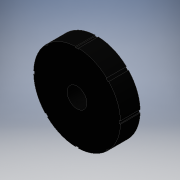
# Autodesk Inventor part: ET2
Saved by Autodesk Inventor 2016 (Build 200138000, 138)
## iProperties
Created: 2016-03-19
Part Number: ET2
Material: Genérico
Document SubType Name: Modeling
Designer: Usuario1
Density: 1 g/cm^3
Appearance: Valor por defecto
Author: Usuario1
Autodesk Inventor part; units mm, degrees
ref_plane "YZ Plane" through (0, 0, 0) normal (1, 0, 0) x (0, 1, 0)
ref_plane "XZ Plane" through (0, 0, 0) normal (0, 1, 0) x (-1, 0, 0)
ref_plane "XY Plane" through (0, 0, 0) normal (0, 0, 1) x (1, 0, 0)
sketch "Boceto1" plane through (0, 0, 0) normal (0, 1, 0) x (-1, 0, 0)
  circle A0 centre (0, 0) radius 0.2442
  circle A1 centre (0, 0) radius 0.28
  line L0 (-0.03, -0.8791) -> (-0.03, -0.8595)
  line L1 (-0.03, -0.8595) -> (0.03, -0.8595)
  line L2 (0.03, -0.8595) -> (0.03, -0.8791)
  line L3 (-0.6428, -0.6004) -> (-0.629, -0.5865)
  line L4 (-0.629, -0.5865) -> (-0.5865, -0.629)
  line L5 (-0.5865, -0.629) -> (-0.6004, -0.6428)
  line L6 (-0.8791, -0.03) -> (-0.8595, -0.03)
  line L7 (-0.8595, -0.03) -> (-0.8595, 0.03)
  line L8 (-0.8595, 0.03) -> (-0.8791, 0.03)
  arc A2 (-0.8791, -0.03) -> (-0.6428, -0.6004) centre (0, 0) ccw
  arc A3 (-0.6004, -0.6428) -> (-0.03, -0.8791) centre (0, 0) ccw
  line L9 (0.03, -0.8791) -> (0.03, -0.8595)
  line L10 (0.03, -0.8595) -> (-0.03, -0.8595)
  line L11 (-0.03, -0.8595) -> (-0.03, -0.8791)
  line L12 (0.6428, -0.6004) -> (0.629, -0.5865)
  line L13 (0.629, -0.5865) -> (0.5865, -0.629)
  line L14 (0.5865, -0.629) -> (0.6004, -0.6428)
  line L15 (0.8791, -0.03) -> (0.8595, -0.03)
  line L16 (0.8595, -0.03) -> (0.8595, 0.03)
  line L17 (0.8595, 0.03) -> (0.8791, 0.03)
  arc A4 (0.6428, -0.6004) -> (0.8791, -0.03) centre (0, 0) ccw
  arc A5 (0.03, -0.8791) -> (0.6004, -0.6428) centre (0, 0) ccw
  line L18 (-0.03, 0.8791) -> (-0.03, 0.8595)
  line L19 (-0.03, 0.8595) -> (0.03, 0.8595)
  line L20 (0.03, 0.8595) -> (0.03, 0.8791)
  line L21 (-0.6428, 0.6004) -> (-0.629, 0.5865)
  line L22 (-0.629, 0.5865) -> (-0.5865, 0.629)
  line L23 (-0.5865, 0.629) -> (-0.6004, 0.6428)
  line L24 (-0.8791, 0.03) -> (-0.8595, 0.03)
  line L25 (-0.8595, 0.03) -> (-0.8595, -0.03)
  line L26 (-0.8595, -0.03) -> (-0.8791, -0.03)
  arc A6 (-0.6428, 0.6004) -> (-0.8791, 0.03) centre (0, 0) ccw
  arc A7 (-0.03, 0.8791) -> (-0.6004, 0.6428) centre (0, 0) ccw
  line L27 (0.03, 0.8791) -> (0.03, 0.8595)
  line L28 (0.03, 0.8595) -> (-0.03, 0.8595)
  line L29 (-0.03, 0.8595) -> (-0.03, 0.8791)
  line L30 (0.6428, 0.6004) -> (0.629, 0.5865)
  line L31 (0.629, 0.5865) -> (0.5865, 0.629)
  line L32 (0.5865, 0.629) -> (0.6004, 0.6428)
  line L33 (0.8791, 0.03) -> (0.8595, 0.03)
  line L34 (0.8595, 0.03) -> (0.8595, -0.03)
  line L35 (0.8595, -0.03) -> (0.8791, -0.03)
  arc A8 (0.8791, 0.03) -> (0.6428, 0.6004) centre (0, 0) ccw
  arc A9 (0.6004, 0.6428) -> (0.03, 0.8791) centre (0, 0) ccw
  circle A10 centre (0, 0) radius 0.2
  point P0 (0, 0)
  constraints: 72 end point, 16 point on circle, 11 centre point
extrude "Extrusión1" add sketch "Boceto1" along normal blind 0.4 contours A0 | A1 | A3 L5 L4 L3 A2 L6 L7 L8 A6 L21 L22 L23 A7 L18 L19 L20 A9 L32 L31 L30 A8 L17 L16 L15 A4 L12 L13 L14 A5 L2 L1 L0
sketch "Boceto2" plane through (0, 0.4, 0) normal (0, 1, 0) x (1, 0, 0)
  circle A0 centre (0, 0) radius 0.2442
  circle A1 centre (0, 0) radius 0.28
  line L0 (-0.03, -0.8791) -> (-0.03, -0.8595)
  line L1 (-0.03, -0.8595) -> (0.03, -0.8595)
  line L2 (0.03, -0.8595) -> (0.03, -0.8791)
  line L3 (-0.6428, -0.6004) -> (-0.629, -0.5865)
  line L4 (-0.629, -0.5865) -> (-0.5865, -0.629)
  line L5 (-0.5865, -0.629) -> (-0.6004, -0.6428)
  line L6 (-0.8791, -0.03) -> (-0.8595, -0.03)
  line L7 (-0.8595, -0.03) -> (-0.8595, 0.03)
  line L8 (-0.8595, 0.03) -> (-0.8791, 0.03)
  arc A2 (-0.8791, -0.03) -> (-0.6428, -0.6004) centre (0, 0) ccw
  arc A3 (-0.6004, -0.6428) -> (-0.03, -0.8791) centre (0, 0) ccw
  line L9 (0.03, -0.8791) -> (0.03, -0.8595)
  line L10 (0.03, -0.8595) -> (-0.03, -0.8595)
  line L11 (-0.03, -0.8595) -> (-0.03, -0.8791)
  line L12 (0.6428, -0.6004) -> (0.629, -0.5865)
  line L13 (0.629, -0.5865) -> (0.5865, -0.629)
  line L14 (0.5865, -0.629) -> (0.6004, -0.6428)
  line L15 (0.8791, -0.03) -> (0.8595, -0.03)
  line L16 (0.8595, -0.03) -> (0.8595, 0.03)
  line L17 (0.8595, 0.03) -> (0.8791, 0.03)
  arc A4 (0.6428, -0.6004) -> (0.8791, -0.03) centre (0, 0) ccw
  arc A5 (0.03, -0.8791) -> (0.6004, -0.6428) centre (0, 0) ccw
  line L18 (-0.03, 0.8791) -> (-0.03, 0.8595)
  line L19 (-0.03, 0.8595) -> (0.03, 0.8595)
  line L20 (0.03, 0.8595) -> (0.03, 0.8791)
  line L21 (-0.6428, 0.6004) -> (-0.629, 0.5865)
  line L22 (-0.629, 0.5865) -> (-0.5865, 0.629)
  line L23 (-0.5865, 0.629) -> (-0.6004, 0.6428)
  line L24 (-0.8791, 0.03) -> (-0.8595, 0.03)
  line L25 (-0.8595, 0.03) -> (-0.8595, -0.03)
  line L26 (-0.8595, -0.03) -> (-0.8791, -0.03)
  arc A6 (-0.6428, 0.6004) -> (-0.8791, 0.03) centre (0, 0) ccw
  arc A7 (-0.03, 0.8791) -> (-0.6004, 0.6428) centre (0, 0) ccw
  line L27 (0.03, 0.8791) -> (0.03, 0.8595)
  line L28 (0.03, 0.8595) -> (-0.03, 0.8595)
  line L29 (-0.03, 0.8595) -> (-0.03, 0.8791)
  line L30 (0.6428, 0.6004) -> (0.629, 0.5865)
  line L31 (0.629, 0.5865) -> (0.5865, 0.629)
  line L32 (0.5865, 0.629) -> (0.6004, 0.6428)
  line L33 (0.8791, 0.03) -> (0.8595, 0.03)
  line L34 (0.8595, 0.03) -> (0.8595, -0.03)
  line L35 (0.8595, -0.03) -> (0.8791, -0.03)
  arc A8 (0.8791, 0.03) -> (0.6428, 0.6004) centre (0, 0) ccw
  arc A9 (0.6004, 0.6428) -> (0.03, 0.8791) centre (0, 0) ccw
  circle A10 centre (0, 0) radius 0.2
  constraints: 72 end point, 16 point on circle, 11 centre point
extrude "Extrusión2" add sketch "Boceto2" along normal blind 0.125 contours A0 | A1
chamfer "Chaflán1" distance 0.04 angle 45 1 edges at (-0.28, 0.525, 0)
sketch "Boceto3" plane through (0, 0, 0) normal (0, -1, 0) x (1, 0, 0)
  circle A0 centre (0, 0) radius 0.2 projected
  circle A1 centre (0, 0) radius 0.2 projected
  line L0 (0.03, -0.8791) -> (0.03, -0.8595) projected
  arc A2 (0.03, -0.8791) -> (0.6004, -0.6428) centre (0, 0) ccw projected
  line L1 (0.5865, -0.629) -> (0.6004, -0.6428) projected
  line L2 (0.629, -0.5865) -> (0.5865, -0.629) projected
  line L3 (0.6428, -0.6004) -> (0.629, -0.5865) projected
  arc A3 (0.6428, -0.6004) -> (0.8791, -0.03) centre (0, 0) ccw projected
  line L4 (0.8595, -0.03) -> (0.8791, -0.03) projected
  line L5 (0.8595, 0.03) -> (0.8595, -0.03) projected
  line L6 (0.8791, 0.03) -> (0.8595, 0.03) projected
  arc A4 (0.8791, 0.03) -> (0.6428, 0.6004) centre (0, 0) ccw projected
  line L7 (0.629, 0.5865) -> (0.6428, 0.6004) projected
  line L8 (0.5865, 0.629) -> (0.629, 0.5865) projected
  line L9 (0.6004, 0.6428) -> (0.5865, 0.629) projected
  arc A5 (0.6004, 0.6428) -> (0.03, 0.8791) centre (0, 0) ccw projected
  line L10 (0.03, 0.8595) -> (0.03, 0.8791) projected
  line L11 (-0.03, 0.8595) -> (0.03, 0.8595) projected
  line L12 (-0.03, 0.8791) -> (-0.03, 0.8595) projected
  arc A6 (-0.03, 0.8791) -> (-0.6004, 0.6428) centre (0, 0) ccw projected
  line L13 (-0.5865, 0.629) -> (-0.6004, 0.6428) projected
  line L14 (-0.629, 0.5865) -> (-0.5865, 0.629) projected
  line L15 (-0.6428, 0.6004) -> (-0.629, 0.5865) projected
  arc A7 (-0.6428, 0.6004) -> (-0.8791, 0.03) centre (0, 0) ccw projected
  line L16 (-0.8595, 0.03) -> (-0.8791, 0.03) projected
  line L17 (-0.8595, -0.03) -> (-0.8595, 0.03) projected
  line L18 (-0.8791, -0.03) -> (-0.8595, -0.03) projected
  arc A8 (-0.8791, -0.03) -> (-0.6428, -0.6004) centre (0, 0) ccw projected
  line L19 (-0.629, -0.5865) -> (-0.6428, -0.6004) projected
  line L20 (-0.5865, -0.629) -> (-0.629, -0.5865) projected
  line L21 (-0.6004, -0.6428) -> (-0.5865, -0.629) projected
  arc A9 (-0.6004, -0.6428) -> (-0.03, -0.8791) centre (0, 0) ccw projected
  line L22 (-0.03, -0.8595) -> (-0.03, -0.8791) projected
  line L23 (0.03, -0.8595) -> (-0.03, -0.8595) projected
  arc A10 (0.7095, 0.1701) -> (0.622, 0.3814) centre (0, 0) ccw
  line L24 (0.7095, 0.1701) -> (0.7095, -0.1701)
  arc A11 (0.622, -0.3814) -> (0.7095, -0.1701) centre (0, 0) ccw
  line L25 (0.622, -0.3814) -> (0.3814, -0.622)
  arc A12 (0.1701, -0.7095) -> (0.3814, -0.622) centre (0, 0) ccw
  line L26 (0.1701, -0.7095) -> (-0.1701, -0.7095)
  arc A13 (-0.3814, -0.622) -> (-0.1701, -0.7095) centre (0, 0) ccw
  line L27 (-0.3814, -0.622) -> (-0.622, -0.3814)
  arc A14 (-0.7095, -0.1701) -> (-0.622, -0.3814) centre (0, 0) ccw
  line L28 (-0.7095, -0.1701) -> (-0.7095, 0.1701)
  arc A15 (-0.622, 0.3814) -> (-0.7095, 0.1701) centre (0, 0) ccw
  line L29 (-0.622, 0.3814) -> (-0.3814, 0.622)
  arc A16 (-0.1701, 0.7095) -> (-0.3814, 0.622) centre (0, 0) ccw
  line L30 (-0.1701, 0.7095) -> (0.1701, 0.7095)
  arc A17 (0.3814, 0.622) -> (0.1701, 0.7095) centre (0, 0) ccw
  line L31 (0.3814, 0.622) -> (0.622, 0.3814)
  circle A18 centre (0, 0) radius 0.35
  point P0 (0, 0)
  dimension "d7" = 0.15
  dimension "d8" = 0.15
  constraints: 16 end point, 16 point on circle, 9 centre point, 15 other
  measures "d7" radial gap between concentric circles of A4 A10
  measures "d8" radial gap between concentric circles of A0 A18
extrude "Extrusión3" cut sketch "Boceto3" against normal blind 0.3 contours L24 A11 L25 A12 L26 A13 L27 A14 L28 A15 L29 A16 L30 A17 L31 A10
sketch "Boceto4" plane through (0, 0, 0) normal (0, -1, 0) x (1, 0, 0)
  circle A0 centre (0, 0) radius 0.35 projected
  arc A1 (0.7095, 0.1701) -> (0.622, 0.3814) centre (0, 0) ccw projected
  line L0 (0.3814, 0.622) -> (0.622, 0.3814) projected
  arc A2 (0.3814, 0.622) -> (0.1701, 0.7095) centre (0, 0) ccw projected
  line L1 (-0.1701, 0.7095) -> (0.1701, 0.7095) projected
  arc A3 (-0.1701, 0.7095) -> (-0.3814, 0.622) centre (0, 0) ccw projected
  line L2 (-0.622, 0.3814) -> (-0.3814, 0.622) projected
  arc A4 (-0.622, 0.3814) -> (-0.7095, 0.1701) centre (0, 0) ccw projected
  line L3 (-0.7095, -0.1701) -> (-0.7095, 0.1701) projected
  arc A5 (-0.7095, -0.1701) -> (-0.622, -0.3814) centre (0, 0) ccw projected
  line L4 (-0.3814, -0.622) -> (-0.622, -0.3814) projected
  arc A6 (-0.3814, -0.622) -> (-0.1701, -0.7095) centre (0, 0) ccw projected
  line L5 (0.1701, -0.7095) -> (-0.1701, -0.7095) projected
  arc A7 (0.1701, -0.7095) -> (0.3814, -0.622) centre (0, 0) ccw projected
  line L6 (0.622, -0.3814) -> (0.3814, -0.622) projected
  arc A8 (0.622, -0.3814) -> (0.7095, -0.1701) centre (0, 0) ccw projected
  line L7 (0.7095, 0.1701) -> (0.7095, -0.1701) projected
  point P0 (0, 0)
extrude "Extrusión4" add sketch "Boceto4" against normal blind 0.15
